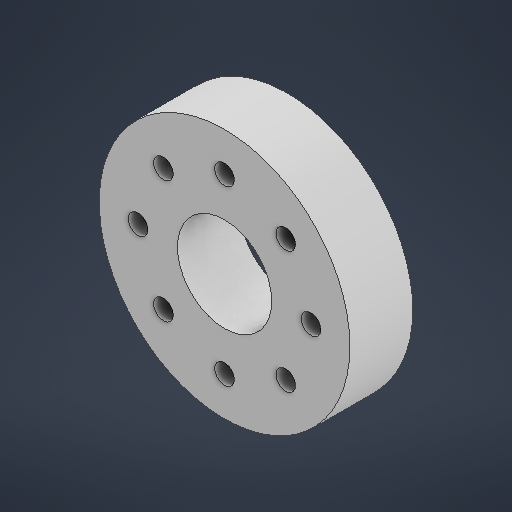
# Autodesk Inventor part: FifthAxisShaft
Saved by Autodesk Inventor 2025 (Build 290162000, 162)
## iProperties
Created: 2024-05-20
Part Number: FifthAxisShaft
Material: Generic
Document SubType Name: Modeling
Designer: avsar
Density: 1 g/cm^3
Appearance: Default
Author: avsar
Autodesk Inventor part; units mm, degrees
ref_plane "YZ Plane" through (0, 0, 0) normal (1, 0, 0) x (0, 1, 0)
ref_plane "XZ Plane" through (0, 0, 0) normal (0, 1, 0) x (-1, 0, 0)
ref_plane "XY Plane" through (0, 0, 0) normal (0, 0, 1) x (1, 0, 0)
sketch "Sketch1" plane through (0, 0, 0) normal (0, 0, 1) x (1, 0, 0)
  circle A0 centre (0, 0) radius 15.95
  circle A1 centre (0, 11) radius 1.25
  circle A2 centre (-7.7782, 7.7782) radius 1.25
  circle A3 centre (-11, 0) radius 1.25
  circle A4 centre (-7.7782, -7.7782) radius 1.25
  circle A5 centre (0, -11) radius 1.25
  circle A6 centre (7.7782, -7.7782) radius 1.25
  circle A7 centre (11, 0) radius 1.25
  circle A8 centre (7.7782, 7.7782) radius 1.25
  circle A9 centre (0, 0) radius 6
  dimension "d0" = 31.9
  dimension "d1" = 2.5
  dimension "d2" = 11
  dimension "d5" = 360
  dimension "d17" = 12
  constraints: 10 centre point, 2 coincident, 1 vertical alignment, 17 other
  measures "d0" diameter of A0
  measures "d1" diameter of A1
  measures "d2" distance of A1.centre point (0, 0)
  measures "d17" diameter of A9
extrude "Extrusion1" add sketch "Sketch1" along normal mid plane 8
body "Solid1"
